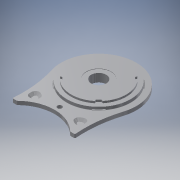
# Autodesk Inventor part: 202-07
Saved by Autodesk Inventor 2019 (Build 230136000, 136)
## iProperties
Company: Autodesk Inc.
Created: 2007-11-01
Part Number: 202-07
Document SubType Name: Modeling
Designer: Autodesk Inc.
Density: 7.85 g/cm^3
Mass: 331.222 g
Surface Area: 155.931 cm^2
Volume: 42.1938 cm^3
Material: Steel
Description: BACK PIVOT PLATE
Appearance: Aluminum - Flat
Component Category: Back Component
Author: Inventor
Autodesk Inventor part; units mm, degrees
ref_plane "XZ Plane" through (0, 0, 0) normal (0, 1, 0) x (-1, 0, 0)
ref_plane "XY Plane" through (0, 0, 0) normal (0, 0, 1) x (1, 0, 0)
sketch "Sketch1" plane through (0, 0, 0) normal (0, 0, 1) x (1, 0, 0)
  arc A0 (39.1735, -12.101) -> (-39.1735, -12.101) centre (0, 0) ccw
  arc A1 (-33.9969, -58.9207) -> (-33, -60) centre (-33, -59) ccw
  arc A2 (33, -60) -> (33.9969, -58.9207) centre (33, -59) ccw
  arc A3 (-33.9969, -58.9207) -> (-39.1735, -12.101) centre (-158.6454, -49.0066) ccw
  line L0 (0, 67) -> (0, -115) projected
  arc A4 (39.1735, -12.101) -> (33.9969, -58.9207) centre (158.6454, -49.0066) ccw
  arc A5 (28.694, -59.7143) -> (-28.694, -59.7143) centre (0, -89) ccw
  line L1 (-29.3939, -60) -> (-33, -60)
  line L2 (33, -60) -> (29.3939, -60)
  arc A6 (28.694, -59.7143) -> (29.3939, -60) centre (29.3939, -59) ccw
  arc A7 (-29.3939, -60) -> (-28.694, -59.7143) centre (-29.3939, -59) ccw
  dimension "d0" = 2
  dimension "d2" = 82
  dimension "d3" = 59
  dimension "d5" = 33
  dimension "d8" = 317.2907
  dimension "d46" = 1
  dimension "d47" = 82
  dimension "d48" = 89
  dimension "d49" = 1
  constraints: 17 point on circle, 9 tangent, 8 centre point, 4 end point, 3 symmetric about line, 1 coincident, 1 collinear, 1 equal radius, 1 perpendicular, 1 point on line, 1 other
  measures "d0" diameter of A1
  measures "d2" diameter of A0
  measures "d3" vertical distance of A1.centre point (0, 0)
  measures "d5" horizontal distance of A1.centre point (0, 0)
  measures "d8" distance of A4.centre A3.centre
  measures "d46" radius of A2
  measures "d47" diameter of A5
  measures "d48" distance of point (0, 0) A5.centre
  measures "d49" radius of A6
extrude "Extrusion1" add sketch "Sketch1" against normal blind 4
sketch "Sketch2" plane through (0, 0, -4) normal (0, 0, -1) x (-1, 0, 0)
  arc A0 (39.1735, -12.101) -> (-39.1735, -12.101) centre (0, 0) ccw projected
  arc A1 (-33.9969, -58.9207) -> (-33, -60) centre (-33, -59) ccw projected
  arc A2 (-23.95, -41.4591) -> (-27.7, -43.6242) centre (-25.2, -43.6242) ccw
  arc A3 (-27.7, -45.8758) -> (-23.95, -48.0409) centre (-25.2, -45.8758) ccw
  arc A4 (-22, -46.9151) -> (-22, -42.5849) centre (-23.25, -44.75) ccw
  line L0 (0, -80.4618) -> (0, 61.2436) projected
  line L1 (33, -60) -> (29.3939, -60) projected
  line L2 (-22, -42.5849) -> (-23.95, -41.4591)
  line L3 (-27.7, -43.6242) -> (-27.7, -45.8758)
  line L4 (-23.95, -48.0409) -> (-22, -46.9151)
  point P0 (-29.1205, 28.8617)
  point P1 (-33.2024, -58.0207)
  point P2 (-4.0693, -52.9372)
  dimension "d15" = 2.5
  dimension "d16" = 23.25
  dimension "d17" = 44.75
  dimension "d19" = 1.95
  dimension "d50" = 60
  dimension "d51" = 60
  constraints: 8 point on circle, 6 end point, 6 tangent, 3 centre point, 2 equal radius, 1 perpendicular
  measures "d15" radius of A2
  measures "d16" horizontal distance of A0.centre A4.centre
  measures "d17" vertical distance of A0.centre A4.centre
  measures "d19" horizontal distance of A2.centre A4.centre
  measures "d50" angle of L0 L4
  measures "d51" angle of L4 L2
extrude "Extrusion2" add sketch "Sketch2" along normal blind 2.5
chamfer "Chamfer1" distance 2.5 angle 45 6 edges at (22.975, -47.478, -4) (26.45, -48.0409, -4) (27.7, -44.75, -4) (26.45, -41.4591, -4) (22.975, -42.022, -4) (20.75, -44.75, -4)
mirror "Mirror1" about plane through (0, 0, 0) normal (1, 0, 0) of "Extrusion2", "Chamfer1"
sketch "Sketch3" plane through (0, 0, 0) normal (0, 0, 1) x (1, 0, 0)
  arc A0 (-22, -46.9151) -> (-22, -42.5849) centre (-23.25, -44.75) ccw projected
  arc A1 (-27.7, -45.8758) -> (-23.95, -48.0409) centre (-25.2, -45.8758) ccw projected
  arc A2 (-23.95, -41.4591) -> (-27.7, -43.6242) centre (-25.2, -43.6242) ccw projected
  line L0 (-23.075, -49.5564) -> (-21.125, -48.4306)
  arc A3 (-21.125, -48.4306) -> (-21.125, -41.0694) centre (-23.25, -44.75) ccw
  line L1 (-21.125, -41.0694) -> (-23.075, -39.9436)
  arc A4 (-23.075, -39.9436) -> (-29.45, -43.6242) centre (-25.2, -43.6242) ccw
  line L2 (-29.45, -43.6242) -> (-29.45, -45.8758)
  arc A5 (-29.45, -45.8758) -> (-23.075, -49.5564) centre (-25.2, -45.8758) ccw
  line L3 (-23.95, -41.4591) -> (-22, -42.5849) projected
  line L4 (-22, -46.9151) -> (-23.95, -48.0409) projected
  line L5 (-27.7, -45.8758) -> (-27.7, -43.6242) projected
  constraints: 6 end point, 6 point on circle, 3 centre point
extrude "Extrusion3" cut sketch "Sketch3" against normal blind 2.5 contours L4 A1 L5 A2 L3 A0 | A5 L2 A4 L1 A3 L0
chamfer "Chamfer2" distance 2.5 angle 45 6 edges at (-27.325, -49.5564, -2.5) (-22.1, -48.9935, -2.5) (-19, -44.75, -2.5) (-22.1, -40.5065, -2.5) (-27.325, -39.9436, -2.5) (-29.45, -44.75, -2.5)
mirror "Mirror2" about plane through (0, 0, 0) normal (1, 0, 0) of "Extrusion3", "Chamfer2"
sketch "Sketch4" plane through (0, 0, 0) normal (0, 0, 1) x (1, 0, 0)
  circle A0 centre (0, 0) radius 8.25
  line L0 (0, 0) -> (0, -42.5)
  circle A1 centre (0, -42.5) radius 2.5
  dimension "d31" = 16.5
  dimension "d32" = 42.5
  dimension "d33" = 5
  constraints: 2 centre point, 2 coincident, 2 end point, 1 vertical
  measures "d31" diameter of A0
  measures "d32" distance of L0.start L0.end
  measures "d33" diameter of A1
extrude "Extrusion4" cut sketch "Sketch4" against normal through all
sketch "Sketch6" plane through (0, 0, 0) normal (0, 1, 0) x (-1, 0, 0)
  line L0 (8.25, -4) -> (8.25, 0) projected
  line L1 (8.25, 0) -> (41, 0) projected
  line L2 (41, 0) -> (41, -4) projected
  line L3 (41, -4) -> (8.25, -4) projected
  line L4 (-8.25, 0) -> (-8.25, -4) projected
  line L5 (-8.25, -4) -> (-41, -4) projected
  line L6 (-41, -4) -> (-41, 0) projected
  line L7 (-41, 0) -> (-8.25, 0) projected
  line L8 (-34.665, 0) -> (-34.665, 3.3)
  line L9 (-34.665, 3.3) -> (-30, 3.3)
  line L10 (-30, 3.3) -> (-30, 5.4)
  line L11 (-30, 5.4) -> (-13.5, 5.4)
  line L12 (-13.5, 5.4) -> (-13.5, 5)
  line L13 (-13.5, 5) -> (-8.25, 5)
  line L14 (-8.25, 5) -> (-8.25, 0)
  line L15 (8.25, 0) -> (41, 0) projected
  line L16 (41, 0) -> (41, -4) projected
  line L17 (41, -4) -> (8.25, -4) projected
  line L18 (-8.25, -4) -> (-41, -4) projected
  line L19 (-41, -4) -> (-41, 0) projected
  line L20 (-41, 0) -> (-8.25, 0) projected
  line L21 (8.25, 0) -> (41, 0) projected
  line L22 (41, 0) -> (41, -4) projected
  line L23 (41, -4) -> (8.25, -4) projected
  line L24 (-8.25, -4) -> (-41, -4) projected
  line L25 (-41, -4) -> (-41, 0) projected
  line L26 (-41, 0) -> (-8.25, 0) projected
  line L27 (8.25, 0) -> (41, 0) projected
  line L28 (41, 0) -> (41, -4) projected
  line L29 (41, -4) -> (8.25, -4) projected
  line L30 (-8.25, -4) -> (-41, -4) projected
  line L31 (-41, -4) -> (-41, 0) projected
  line L32 (-41, 0) -> (-8.25, 0) projected
  line L33 (8.25, 0) -> (41, 0) projected
  line L34 (41, 0) -> (41, -4) projected
  line L35 (41, -4) -> (8.25, -4) projected
  line L36 (-8.25, -4) -> (-41, -4) projected
  line L37 (-41, -4) -> (-41, 0) projected
  line L38 (-41, 0) -> (-8.25, 0) projected
  line L39 (8.25, 0) -> (41, 0) projected
  line L40 (41, 0) -> (41, -4) projected
  line L41 (41, -4) -> (8.25, -4) projected
  line L42 (-8.25, -4) -> (-41, -4) projected
  line L43 (-41, -4) -> (-41, 0) projected
  line L44 (-41, 0) -> (-8.25, 0) projected
  line L45 (0, -5.88) -> (0, 7.28) projected
  line L46 (8.25, -4) -> (8.25, 0) projected
  line L47 (-8.25, 0) -> (-8.25, -4) projected
  line L48 (8.25, -4) -> (8.25, 0) projected
  line L49 (-8.25, 0) -> (-8.25, -4) projected
  line L50 (8.25, -4) -> (8.25, 0) projected
  line L51 (-8.25, 0) -> (-8.25, -4) projected
  line L52 (8.25, -4) -> (8.25, 0) projected
  line L53 (-8.25, 0) -> (-8.25, -4) projected
  line L54 (8.25, -4) -> (8.25, 0) projected
  line L55 (-8.25, 0) -> (-8.25, -4) projected
  point P0 (0, 0)
  dimension "d52" = 5
  dimension "d53" = 5.4
  dimension "d54" = 3.3
  dimension "d55" = 34.665
  dimension "d56" = 30
  dimension "d57" = 13.5
  constraints: 14 end point, 6 parallel, 2 perpendicular, 1 point on line
  measures "d52" distance of L13.end L4.start
  measures "d53" distance between parallel lines of L7 L11
  measures "d54" distance between parallel lines of L7 L9
  measures "d55" distance from line of point (0, 0) L8
  measures "d56" distance from line of point (0, 0) L10
  measures "d57" distance from line of point (0, 0) L12
revolve "Revolution1" add sketch "Sketch6" angle 360 about axis through (0, 0, 0) along (0, 0, 1) contours L7 L8 L9 L10 L11 L12 L13 L14
ref_plane "Work Plane1" through (0, 0, 0) normal (0.7071068, 0.7071068, 0) x (0, 0, 1)
sketch "Sketch7" plane through (0, 0, 0) normal (0.7071068, 0.7071068, 0) x (0, 0, 1)
  line L0 (3.3, -34.665) -> (0, -34.665) projected
  line L1 (0, -34.665) -> (0, -41) projected
  line L2 (0, -41) -> (-4, -41) projected
  line L3 (-4, -41) -> (-4, -8.25) projected
  line L4 (-4, -8.25) -> (5, -8.25) projected
  line L5 (5, -8.25) -> (5, -13.5) projected
  line L6 (5, -13.5) -> (5.4, -13.5) projected
  line L7 (5.4, -13.5) -> (5.4, -30) projected
  line L8 (5.4, -30) -> (3.3, -30) projected
  line L9 (3.3, -30) -> (3.3, -34.665) projected
  line L10 (0, 34.665) -> (3.3, 34.665) projected
  line L11 (3.3, 34.665) -> (3.3, 30) projected
  line L12 (3.3, 30) -> (5.4, 30) projected
  line L13 (5.4, 30) -> (5.4, 13.5) projected
  line L14 (5.4, 13.5) -> (5, 13.5) projected
  line L15 (5, 13.5) -> (5, 8.25) projected
  line L16 (5, 8.25) -> (-4, 8.25) projected
  line L17 (-4, 8.25) -> (-4, 48.7239) projected
  line L18 (-4, 48.7239) -> (0, 48.7239) projected
  line L19 (0, 48.7239) -> (0, 34.665) projected
  line L20 (0, 35.665) -> (1, 34.665)
  line L21 (3.3, -34.665) -> (0, -34.665) projected
  line L22 (0, -34.665) -> (0, -41) projected
  line L23 (0, -41) -> (-4, -41) projected
  line L24 (-4, -41) -> (-4, -8.25) projected
  line L25 (5, -8.25) -> (5, -13.5) projected
  line L26 (5, -13.5) -> (5.4, -13.5) projected
  line L27 (5.4, -13.5) -> (5.4, -30) projected
  line L28 (5.4, -30) -> (3.3, -30) projected
  line L29 (3.3, -30) -> (3.3, -34.665) projected
  line L30 (0, 34.665) -> (3.3, 34.665) projected
  line L31 (3.3, 34.665) -> (3.3, 30) projected
  line L32 (3.3, 30) -> (5.4, 30) projected
  line L33 (5.4, 30) -> (5.4, 13.5) projected
  line L34 (5.4, 13.5) -> (5, 13.5) projected
  line L35 (5, 13.5) -> (5, 8.25) projected
  line L36 (-4, 8.25) -> (-4, 48.7239) projected
  line L37 (-4, 48.7239) -> (0, 48.7239) projected
  line L38 (0, 48.7239) -> (0, 34.665) projected
  line L39 (3.3, -34.665) -> (0, -34.665) projected
  line L40 (0, -34.665) -> (0, -41) projected
  line L41 (0, -41) -> (-4, -41) projected
  line L42 (-4, -41) -> (-4, -8.25) projected
  line L43 (5, -8.25) -> (5, -13.5) projected
  line L44 (5, -13.5) -> (5.4, -13.5) projected
  line L45 (5.4, -13.5) -> (5.4, -30) projected
  line L46 (5.4, -30) -> (3.3, -30) projected
  line L47 (3.3, -30) -> (3.3, -34.665) projected
  line L48 (0, 34.665) -> (3.3, 34.665) projected
  line L49 (3.3, 34.665) -> (3.3, 30) projected
  line L50 (3.3, 30) -> (5.4, 30) projected
  line L51 (5.4, 30) -> (5.4, 13.5) projected
  line L52 (5.4, 13.5) -> (5, 13.5) projected
  line L53 (5, 13.5) -> (5, 8.25) projected
  line L54 (-4, 8.25) -> (-4, 48.7239) projected
  line L55 (-4, 48.7239) -> (0, 48.7239) projected
  line L56 (0, 48.7239) -> (0, 34.665) projected
  line L57 (-5.88, 0) -> (7.28, 0) projected
  line L58 (-4, -8.25) -> (5, -8.25) projected
  line L59 (5, 8.25) -> (-4, 8.25) projected
  line L60 (-4, -8.25) -> (5, -8.25) projected
  line L61 (5, 8.25) -> (-4, 8.25) projected
  point P0 (0, 0)
  dimension "d60" = 35.665
  dimension "d61" = 45
  constraints: 2 end point, 2 point on line
  measures "d60" distance of L20.start point (0, 0)
  measures "d61" angle of L19 L20
revolve "Revolution2" add sketch "Sketch7" angle 17.5 mid plane about axis through (0, 0, 0) along (0, 0, 1) contours L19 L20 L10
pattern_circular "Circular Pattern2" count 4 over 360 about axis through (0, 0, 0) along (0, 0, -1) of "Revolution2"
sketch "Sketch8" plane through (0, 0, 5.4) normal (0, 0, 1) x (1, 0, 0)
  circle A0 centre (0, 0) radius 30 projected
  line L0 (0, 0) -> (21.2132, -21.2132) construction
  line L1 (0, 61.2) -> (0, -80.2) construction
  line L2 (17.9901, -21.4559) -> (19.2757, -22.988)
  line L3 (21.4559, -17.9901) -> (22.988, -19.2757)
  arc A1 (17.9901, -21.4559) -> (21.4559, -17.9901) centre (0, 0) ccw
  arc A2 (0, 28) -> (0, -28) centre (0, 0) ccw
  point P0 (19.799, -19.799)
  dimension "d66" = 45
  dimension "d70" = 10
  dimension "d71" = 5
  dimension "d72" = 28
  dimension "d73" = 5.25
  constraints: 8 point on circle, 6 end point, 3 point on line, 2 centre point, 1 coincident
  measures "d66" angle of L1 L0
  measures "d70" angle of L3 L2
  measures "d71" angle of L0 L3
  measures "d72" radius of A1
  measures "d73" distance of L3.end L2.end
extrude "Extrusion6" cut sketch "Sketch8" against normal up to surface (2.1 mm away) contours L2 A1 L3 A0 picked at (20.5402, -20.9257)
fillet "Fillet2" radius 0.95 4 edges at (21.4559, -17.9901, 4.35) (22.988, -19.2757, 4.35) (17.9901, -21.4559, 4.35) (19.2757, -22.988, 4.35)
pattern_circular "Circular Pattern3" count 4 over 360 about axis through (0, 0, 0) along (0, 0, -1) of "Extrusion6", "Fillet2"
fillet "Fillet3" radius 0.25 5 edges at (0, -34.665, 0) (32.9449, 10.784, 0) (32.9449, -10.784, 0) (-34.665, 0, 0) (0, 34.665, 0)
equation "\"d68\" = d67"
equation "\"d67\" = 5deg"
body "Solid1"
